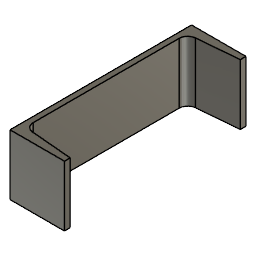
C-300×90×9×13 (Autodesk Fusion 360 design; units mm, degrees)
Autodesk Fusion 360 part; units mm, degrees
note: some values were not read from the file. Set by a fixed rule: which sketch regions a step uses.
sketch "スケッチ1" plane through (0, 0, 0) normal (0, 0, 1) x (1, 0, 0)
  line L0 (0, 0) -> (90, 0)
  line L1 (21.7798, 15.4252) -> (90, 9.4567)
  line L2 (90, 290.5433) -> (21.7798, 284.5748)
  line L3 (0, 300) -> (90, 300)
  line L4 (9, 270.6281) -> (9, 29.3719)
  line L5 (0, 300) -> (0, 0)
  arc A0 (9, 29.3719) -> (21.7798, 15.4252) centre (23, 29.3719) ccw
  arc A1 (21.7798, 284.5748) -> (9, 270.6281) centre (23, 270.6281) ccw
  line L6 (90, 9.4567) -> (90, 0)
  line L7 (90, 300) -> (90, 290.5433)
extrude "押し出し1" add sketch "スケッチ1" along normal blind 100
